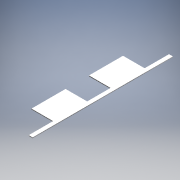
# Autodesk Inventor part: Bottom Mounting Plate
Saved by Autodesk Inventor 2019.4 (Build 234330000, 330)
## iProperties
Created: 2019-12-08
Part Number: Bottom Mounting Plate
Material: Polycarbonate, Smoke
Document SubType Name: Modeling
Designer: admin
Density: 1.2 g/cm^3
Appearance: Polycarbonate - Smoked
Mass: 1665.65 g
Surface Area: 7049.8 cm^2
Volume: 1388.04 cm^3
Author: admin
Autodesk Inventor part; units mm, degrees
ref_plane "YZ Plane" through (0, 0, 0) normal (1, 0, 0) x (0, 1, 0)
ref_plane "XZ Plane" through (0, 0, 0) normal (0, 1, 0) x (-1, 0, 0)
ref_plane "XY Plane" through (0, 0, 0) normal (0, 0, 1) x (1, 0, 0)
sketch "Sketch1" plane through (0, 0, 0) normal (0, 1, 0) x (-1, 0, 0)
  line L0 (-214, 360) -> (214, 360)
  line L1 (214, 360) -> (214, -360)
  line L2 (214, -360) -> (-214, -360)
  line L3 (-214, -360) -> (-214, 360)
  line L4 (-214, 360) -> (214, -360) construction
  line L5 (214, 360) -> (-214, -360) construction
  line L6 (214, -235) -> (325, -235)
  line L7 (325, -235) -> (325, -60)
  line L8 (325, -60) -> (214, -60)
  line L9 (214, -60) -> (214, -235)
  line L10 (214, 60) -> (325, 60)
  line L11 (325, 60) -> (325, 235)
  line L12 (325, 235) -> (214, 235)
  line L13 (214, 235) -> (214, 60)
  line L14 (0, 360) -> (0, 260) construction
  line L15 (0, 360) -> (100, 360) construction
  line L16 (-214, -235) -> (-325, -235)
  line L17 (-325, -235) -> (-325, -60)
  line L18 (-325, -60) -> (-214, -60)
  line L19 (-214, 60) -> (-325, 60)
  line L20 (-325, 60) -> (-325, 235)
  line L21 (-325, 235) -> (-214, 235)
  line L22 (-214, 235) -> (-214, 60)
  line L23 (-214, -60) -> (-214, -235)
  point P0 (0, 0)
  dimension "d0" = 720
  dimension "d1" = 428
  dimension "d4" = 111
  dimension "d5" = 175
  dimension "d6" = 125
  dimension "d7" = 111
  dimension "d8" = 175
  dimension "d9" = 125
  dimension "d10" = 100
  dimension "d11" = 90
  constraints: 48 end point, 8 symmetric about line, 6 parallel, 4 horizontal, 4 perpendicular, 3 midpoint, 2 collinear, 2 point on line, 1 vertical
  measures "d0" distance of L0.end L1.end
  measures "d1" distance of L0.start L0.end
  measures "d4" distance of L8.end L7.end
  measures "d5" distance of L7.end L6.end
  measures "d6" distance between parallel lines of L2 L6
  measures "d7" distance of L12.end L11.end
  measures "d8" distance of L11.end L10.end
  measures "d9" distance between parallel lines of L0 L12
  measures "d10" distance of L14.start L14.end
  measures "d11" angle of L14 L15
extrude "Extrusion1" add sketch "Sketch1" along normal blind 2
fillet "Fillet1" radius 50 8 edges at (214, 1, -235) (214, 1, -60) (214, 1, 60) (214, 1, 235) (-214, 1, 60) (-214, 1, -60) (-214, 1, -235) (-214, 1, 235)
body "Solid1"
